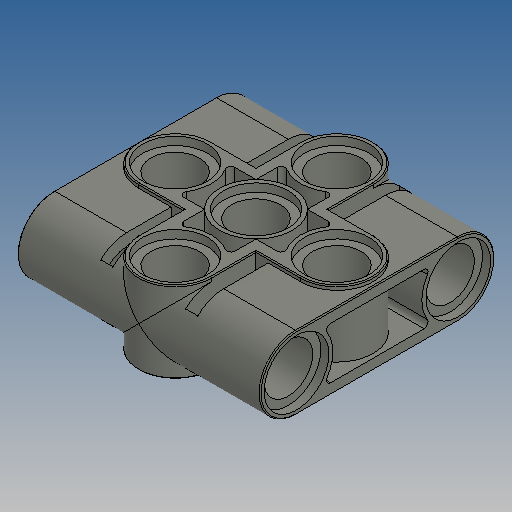
# Autodesk Inventor part: 39793-DkBluishGray
Saved by Autodesk Inventor 2025 (Build 290162010, 162A)
## iProperties
Created: 2020-06-03
Part Number: 39793-DkBluishGray
Material: ABS Plastic
Document SubType Name: Modeling
Designer: D. Kohfeld
Density: 1.06 g/cm^3
Appearance: DkBluishGray
Author: D. Kohfeld
Autodesk Inventor part; units mm, degrees
ref_plane "YZ Plane" through (0, 0, 0) normal (1, 0, 0) x (0, 1, 0)
ref_plane "XZ Plane" through (0, 0, 0) normal (0, 1, 0) x (-1, 0, 0)
ref_plane "XY Plane" through (0, 0, 0) normal (0, 0, 1) x (1, 0, 0)
sketch "Sketch2" plane through (0, 0, 0) normal (1, 0, 0) x (0, 1, 0)
  line L0 (-3.6, 8) -> (-3.6, -8)
  arc A0 (-3.6, -8) -> (3.6, -8) centre (0, -8) ccw
  line L1 (3.6, -8) -> (3.6, 8)
  arc A1 (3.6, 8) -> (-3.6, 8) centre (0, 8) ccw
  line L2 (-2.5456, 5.4544) -> (-2.5456, -5.4544)
  line L3 (2.5456, -5.4544) -> (2.5456, 5.4544)
  arc A2 (-2.5456, 5.4544) -> (2.5456, 5.4544) centre (0, 8) ccw
  arc A3 (2.5456, -5.4544) -> (-2.5456, -5.4544) centre (0, -8) ccw
  line L4 (-2.5456, 5.4544) -> (0, 8) construction
  point P0 (0, 0)
  point P1 (-3.6, 0)
  dimension "d2" = 16
  dimension "d3" = 7.2
  dimension "d4" = 45
  constraints: 10 end point, 8 point on circle, 4 centre point, 4 tangent, 4 vertical, 2 coincident, 2 concentric, 2 horizontal alignment, 1 midpoint, 1 vertical alignment
  measures "d2" distance of A0.centre A1.centre
  measures "d3" distance between parallel lines of L0 L1
  measures "d4" angle of L0 L4
extrude "Extrusion1" add sketch "Sketch2" along normal mid plane 24
sketch "Sketch3" plane through (0, 0, 0) normal (0, 1, 0) x (-1, 0, 0)
  circle A0 centre (0, 0) radius 2.4
  circle A1 centre (0, 0) radius 3.2
  line L0 (12, 11.6) -> (-12, 11.6) construction
  line L1 (12, -11.6) -> (-12, -11.6) construction
  circle A2 centre (0, 8) radius 3.2
  circle A3 centre (0, 8) radius 2.4
  circle A4 centre (-8, 0) radius 3.2
  circle A5 centre (-8, 0) radius 2.4
  circle A6 centre (8, 0) radius 2.4
  circle A7 centre (8, 0) radius 3.2
  circle A8 centre (0, -8) radius 3.2
  circle A9 centre (0, -8) radius 2.4
  line L2 (0, 8) -> (0, 0) construction
  line L3 (0, 0) -> (0, -8) construction
  line L4 (0, 0) -> (-8, 0) construction
  line L5 (0, 0) -> (8, 0) construction
  line L6 (-8, 3.6) -> (-3.6, 3.6)
  line L7 (-3.6, 3.6) -> (-3.6, 8)
  arc A10 (3.6, 8) -> (-3.6, 8) centre (0, 8) ccw
  line L8 (3.6, 8) -> (3.6, 3.6)
  line L9 (3.6, 3.6) -> (8, 3.6)
  arc A11 (8, -3.6) -> (8, 3.6) centre (8, 0) ccw
  line L10 (8, -3.6) -> (3.6, -3.6)
  line L11 (3.6, -3.6) -> (3.6, -8)
  arc A12 (-3.6, -8) -> (3.6, -8) centre (0, -8) ccw
  line L12 (-3.6, -8) -> (-3.6, -3.6)
  line L13 (-3.6, -3.6) -> (-8, -3.6)
  arc A13 (-8, 3.6) -> (-8, -3.6) centre (-8, 0) ccw
  circle A14 centre (0, 0) radius 3.6
  line L14 (-2.5456, 2.5456) -> (-2.5456, 5.4544)
  line L15 (-2.5456, 2.5456) -> (-5.4544, 2.5456)
  line L16 (-5.4544, -2.5456) -> (-2.5456, -2.5456)
  line L17 (-2.5456, -2.5456) -> (-2.5456, -5.4544)
  line L18 (2.5456, -5.4544) -> (2.5456, -2.5456)
  line L19 (2.5456, -2.5456) -> (5.4544, -2.5456)
  line L20 (5.4544, 2.5456) -> (2.5456, 2.5456)
  line L21 (2.5456, 2.5456) -> (2.5456, 5.4544)
  arc A15 (-2.5456, 5.4544) -> (2.5456, 5.4544) centre (0, 8) ccw
  arc A16 (-5.4544, -2.5456) -> (-5.4544, 2.5456) centre (-8, 0) ccw
  arc A17 (2.5456, -5.4544) -> (-2.5456, -5.4544) centre (0, -8) ccw
  arc A18 (5.4544, 2.5456) -> (5.4544, -2.5456) centre (8, 0) ccw
  line L22 (-3.6, -3.6) -> (-4.8, -3.6)
  line L23 (-4.8, -3.6) -> (-4.8, -10.546)
  line L24 (-4.8, -10.546) -> (-3.6, -10.546)
  line L25 (-3.6, -10.546) -> (-3.6, -3.6)
  line L26 (3.6, -3.6) -> (4.8, -3.6)
  line L27 (4.8, -3.6) -> (4.8, -10.546)
  line L28 (4.8, -10.546) -> (3.6, -10.546)
  line L29 (3.6, -10.546) -> (3.6, -3.6)
  line L30 (3.6, 3.6) -> (4.8, 3.6)
  line L31 (4.8, 3.6) -> (4.8, 10.546)
  line L32 (4.8, 10.546) -> (3.6, 10.546)
  line L33 (3.6, 10.546) -> (3.6, 3.6)
  line L34 (-3.6, 3.6) -> (-4.8, 3.6)
  line L35 (-4.8, 3.6) -> (-4.8, 10.546)
  line L36 (-4.8, 10.546) -> (-3.6, 10.546)
  line L37 (-3.6, 10.546) -> (-3.6, 3.6)
  dimension "d7" = 7.2
  dimension "d8" = 4.8
  dimension "d9" = 6.4
  dimension "d14" = 1.2
  dimension "d15" = 2.546
  constraints: 72 end point, 20 point on circle, 19 centre point, 16 equal radius, 14 coincident, 14 horizontal, 12 equal length, 10 tangent, 10 vertical, 8 parallel, 4 perpendicular, 1 concentric, 1 horizontal alignment, 1 point on line
  measures "d7" distance between parallel lines of L8 L7
  measures "d8" diameter of A3
  measures "d9" diameter of A2
  measures "d14" distance of L35.end L36.end
  measures "d15" distance from line of L36 A2.centre
extrude "Extrusion3" cut sketch "Sketch3" along normal through all both and the other way through all contours A0 | A1 | A2 | A3 | A4 | A5 | A6 | A7 | A8 | A9 | L35 L36 L37 L7 L6 | L13 L12 L25 L24 L23 | L33 L32 L31 L9 L8 | L11 L10 L27 L28 L29 | A14 L20 A18 L19 | A14 L14 A15 L21 | L18 A17 L17 A14 | A14 L16 A16 L15
extrude "Extrusion2" add sketch "Sketch3" along normal mid plane 8 contours L6 L7 A10 L8 L9 A11 L10 L11 A12 L12 L13 A13
extrude "Extrusion4" add sketch "Sketch3" along normal mid plane 8 contours A14
extrude "Extrusion5" add sketch "Sketch3" along normal mid plane 6.4 contours A1 | A2 | A4 | A7 | A8
extrude "Extrusion8" add sketch "Sketch3" along normal mid plane 1.6 contours A14 L20 A18 L19 | A14 L14 A15 L21 | L18 A17 L17 A14 | A14 L16 A16 L15
sketch "Sketch4" plane through (12, 0, 0) normal (1, 0, 0) x (0, 0, -1)
  arc A0 (8, -3.6) -> (8, 3.6) centre (8, 0) ccw construction
  arc A1 (-8, 3.6) -> (-8, -3.6) centre (-8, 0) ccw construction
  circle A2 centre (-8, 0) radius 3.2
  circle A3 centre (-8, 0) radius 2.4
  circle A4 centre (8, 0) radius 3.2
  circle A5 centre (8, 0) radius 2.4
  point P0 (0, 0)
  dimension "d20" = 4.8
  dimension "d21" = 6.4
  constraints: 4 centre point, 4 coincident, 2 equal radius
  measures "d20" diameter of A3
  measures "d21" diameter of A2
extrude "Extrusion6" cut sketch "Sketch4" against normal blind 8 contours A3 | A5
extrude "Extrusion7" cut sketch "Sketch4" against normal blind 0.8
mirror "Mirror1" about plane through (0, 0, 0) normal (1, 0, 0) of "Extrusion6", "Extrusion7"
fillet "Fillet1" radius 0.1 32 edges at (0, 4, 11.6) (3.6, 4, 5.8) (-3.6, 4, 5.8) (-11.6, 4, 0) (-5.8, 4, -3.6) (-5.8, 4, 3.6) (0, 4, -11.6) (3.6, 4, -5.8) (-3.6, 4, -5.8) (11.6, 4, 0) (5.8, 4, 3.6) (5.8, 4, -3.6) (12, 0, 11.6) (12, -3.6, 0) (12, 0, -11.6) (12, 3.6, 0) (-12, 0, -11.6) (-12, -3.6, 0) (-12, 0, 11.6) (-12, 3.6, 0) (0, -4, -11.6) (3.6, -4, -5.8) (-3.6, -4, -5.8) (-11.6, -4, 0) (-5.8, -4, 3.6) (-5.8, -4, -3.6) (0, -4, 11.6) (3.6, -4, 5.8) (-3.6, -4, 5.8) (11.6, -4, 0) (5.8, -4, -3.6) (5.8, -4, 3.6)
fillet "Fillet1" radius 0.4 24 edges at (-5.4544, -2.4, 2.5456) (-5.4544, -2.4, -2.5456) (-2.5456, -2.4, -5.4544) (2.5456, -2.4, -5.4544) (5.4544, -2.4, -2.5456) (5.4544, -2.4, 2.5456) (2.5456, -2.4, 5.4544) (-2.5456, -2.4, 5.4544) (-8.4, 2.5456, 5.4544) (-8.4, -2.5456, -5.4544) (-8.4, 2.5456, -5.4544) (-8.4, -2.5456, 5.4544) (8.4, 2.5456, 5.4544) (8.4, -2.5456, 5.4544) (8.4, -2.5456, -5.4544) (8.4, 2.5456, -5.4544) (-5.4544, 2.4, 2.5456) (-5.4544, 2.4, -2.5456) (-2.5456, 2.4, -5.4544) (2.5456, 2.4, -5.4544) (5.4544, 2.4, -2.5456) (5.4544, 2.4, 2.5456) (2.5456, 2.4, 5.4544) (-2.5456, 2.4, 5.4544)
equation "\"d2\" = 2 * lu"
equation "\"d3\" = tlad"
equation "\"d5\" = 3 * lu"
equation "\"d7\" = tlad"
equation "\"d8\" = tpd"
equation "\"d9\" = tsd"
equation "\"d10\" = lu"
equation "\"d16\" = lu"
equation "\"d18\" = lu - 2 * tsl"
equation "\"d26\" = wall"
equation "\"d20\" = tpd"
equation "\"d21\" = tsd"
equation "\"d22\" = lu"
equation "\"d24\" = tsl"
equation "\"d28\" = lf"
equation "\"d29\" = tf"
equation "\"lu\" = 8"
equation "\"tlad\" = 7.2"
equation "\"tpd\" = 4.8"
equation "\"tsd\" = 6.4"
equation "\"tsl\" = 0.8"
equation "\"wall\" = 1.6"
equation "\"lf\" = 0.1"
equation "\"tf\" = 0.4"
body "Solid1"
